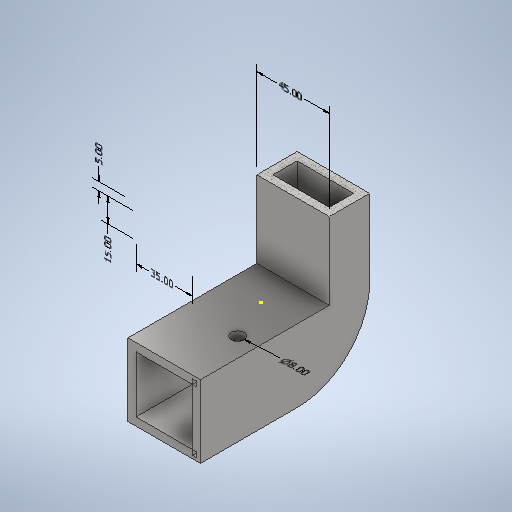
# Autodesk Inventor part: Part2
Saved by Autodesk Inventor 2025.4 (Build 294407000, 407)
## iProperties
Created: 2026-03-03
Part Number: Part2
Material: Iron, Malleable
Document SubType Name: Modeling
Designer: Amir
Density: 7.15 g/cm^3
Appearance: Semi-Polished
Author: Amir
Autodesk Inventor part; units mm, degrees
ref_plane "YZ Plane" through (0, 0, 0) normal (1, 0, 0) x (0, 1, 0)
ref_plane "XZ Plane" through (0, 0, 0) normal (0, 1, 0) x (-1, 0, 0)
ref_plane "XY Plane" through (0, 0, 0) normal (0, 0, 1) x (1, 0, 0)
sketch "Sketch1" plane through (0, 0, 0) normal (0, 0, 1) x (1, 0, 0)
  line L0 (-22.5, -22.5) -> (22.5, -22.5)
  line L1 (22.5, -22.5) -> (22.5, 22.5)
  line L2 (22.5, 22.5) -> (-22.5, 22.5)
  line L3 (-22.5, 22.5) -> (-22.5, -22.5)
  line L4 (-22.5, -22.5) -> (22.5, 22.5) construction
  line L5 (22.5, -22.5) -> (-22.5, 22.5) construction
  line L6 (-17.5, -17.5) -> (17.5, -17.5)
  line L7 (17.5, -17.5) -> (17.5, 17.5)
  line L8 (17.5, 17.5) -> (-17.5, 17.5)
  line L9 (-17.5, 17.5) -> (-17.5, -17.5)
  line L10 (-17.5, -17.5) -> (17.5, 17.5) construction
  line L11 (17.5, -17.5) -> (-17.5, 17.5) construction
  line L12 (-22.5, 17.5) -> (22.5, 17.5)
  point P0 (0, 0)
  dimension "d0" = 45
  dimension "d20" = 5
  dimension "d21" = 5
  constraints: 26 end point, 4 midpoint, 4 parallel, 4 point on line, 2 horizontal, 2 perpendicular
  measures "d0" distance of L2.end L1.end
  measures "d20" distance between parallel lines of L2 L8
  measures "d21" distance between parallel lines of L1 L7
extrude "Extrusion1" add sketch "Sketch1" along normal blind 60 contours L3 L12 L9 L6 L7 L1 L0 | L3 L2 L1 L12 L8
sketch "Sketch2" plane through (0, 0, 0) normal (0, 0, -1) x (-1, 0, 0)
  line L0 (17.5, -17.5) -> (17.5, 17.5) projected
  line L1 (-17.5, -17.5) -> (17.5, -17.5)
  line L2 (17.5, -17.5) -> (17.5, 17.5)
  line L3 (17.5, 17.5) -> (-17.5, 17.5)
  line L4 (-17.5, 17.5) -> (-17.5, -17.5)
  line L5 (-17.5, -17.5) -> (17.5, 17.5) construction
  line L6 (17.5, -17.5) -> (-17.5, 17.5) construction
  line L7 (-22.5, 22.5) -> (22.5, 22.5) projected
  line L8 (-22.5, -22.5) -> (22.5, -22.5)
  line L9 (22.5, -22.5) -> (22.5, 22.5)
  line L10 (22.5, 22.5) -> (-22.5, 22.5)
  line L11 (-22.5, 22.5) -> (-22.5, -22.5)
  line L12 (-22.5, -22.5) -> (22.5, 22.5) construction
  line L13 (22.5, -22.5) -> (-22.5, 22.5) construction
  line L14 (-39.1057, 22.5) -> (57.4203, 22.5)
  point P0 (0, 0)
  dimension "d18" = 5
  dimension "d19" = 5
  constraints: 26 end point, 4 midpoint, 4 parallel, 2 horizontal, 2 perpendicular, 1 point on line
  measures "d18" distance between parallel lines of L8 L1
  measures "d19" distance between parallel lines of L11 L4
revolve "Revolution1" add sketch "Sketch2" angle 90 about axis through (39.1057, 22.5, 0) along (1, 0, 0)
sketch "Sketch3" plane through (-22.5, 22.5, 60) normal (0, 1, 0) x (1, 0, 0)
  line L0 (5, 65) -> (5, 100) projected
  line L1 (40, 85) -> (5, 85)
  line L2 (5, 85) -> (5, 100)
  line L3 (5, 100) -> (40, 100)
  line L4 (35.2339, 98.1928) -> (5, 100) construction
  line L5 (5, 85) -> (35.2339, 113.1928) construction
  line L6 (0, 60) -> (0, 105) projected
  line L7 (45, 80) -> (0, 80)
  line L8 (0, 80) -> (0, 105)
  line L9 (0, 105) -> (45, 105)
  line L10 (40.2339, 93.1928) -> (0, 105) construction
  line L11 (0, 80) -> (45, 122.7171) construction
  line L12 (40, 100) -> (40, 65) projected
  line L13 (40, 100) -> (40, 85)
  line L14 (45, 105) -> (45, 0) projected
  line L15 (45, 105) -> (45, 80)
  point P0 (22.5, 60)
  point P1 (20.117, 99.0964)
  point P2 (43.816, 121.1954)
  point P3 (20.117, 99.0964)
  point P4 (0, 80)
  point P5 (5, 85)
  dimension "d17" = 15
  constraints: 24 end point, 7 point on line, 4 midpoint, 2 horizontal, 2 parallel, 2 perpendicular
  measures "d17" distance between parallel lines of L3 L1
extrude "Extrusion2" add sketch "Sketch3" along normal blind 50
extrude "Extrusion4" add sketch "Sketch1" against normal blind 25 contours L3 L2 L1 L12 L8
extrude "Extrusion5" cut sketch "Sketch3" along normal blind 75.5 contours L0 L3 L12 L1
sketch "Sketch10" plane through (-22.5, 72.5, 60) normal (0, 1, 0) x (1, 0, 0)
  line L0 (45, 105) -> (0, 105)
  line L1 (0, 105) -> (0, 80)
  line L2 (0, 80) -> (45, 80)
  line L3 (45, 80) -> (45, 105)
  line L4 (5, 100) -> (40, 100) projected
  line L5 (40, 85) -> (5, 85) projected
  line L6 (40, 100) -> (5, 100)
  line L7 (5, 100) -> (5, 85)
  line L8 (5, 85) -> (40, 85)
  line L9 (40, 85) -> (40, 100)
  line L10 (-3.6161, 80) -> (47.5585, 80)
  constraints: 18 end point, 4 parallel, 2 horizontal, 2 perpendicular, 1 point on line
revolve "Revolution3" add sketch "Sketch10" angle 90 about axis through (-26.1161, 72.5, -20) along (1, 0, 0)
sketch "Sketch11" plane through (-22.5, 22.5, -20) normal (0, 0, 1) x (1, 0, 0)
  line L0 (45, 75) -> (0, 75) projected
  line L1 (45, 50) -> (0, 50) projected
  line L2 (45, 75) -> (0, 75)
  line L3 (0, 75) -> (0, 50)
  line L4 (0, 50) -> (45, 50)
  line L5 (45, 50) -> (45, 75)
  line L6 (40, 70) -> (40, 55) projected
  line L7 (40, 55) -> (5, 55) projected
  line L8 (40, 70) -> (5, 70)
  line L9 (5, 70) -> (5, 55)
  line L10 (5, 55) -> (40, 55)
  line L11 (40, 55) -> (40, 70)
  point P0 (22.5, -22.5)
  dimension "d68" = 15
  constraints: 16 end point, 4 parallel, 2 horizontal, 2 perpendicular
  measures "d68" distance between parallel lines of L7 L8
extrude "Extrusion8" add sketch "Sketch11" along normal blind 80
sketch "Sketch12" plane through (-22.5, 22.5, 60) normal (0, 1, 0) x (1, 0, 0)
  point P0 (22.5, 60)
sketch "Sketch13" plane through (0, 0, 60) normal (0, 0, 1) x (1, 0, 0)
  line L0 (17.5, 17.5) -> (17.5, -17.5) projected
  line L1 (17.5, 17.5) -> (19.8638, 17.5)
  line L2 (19.8638, 17.5) -> (19.8638, 20.41)
  line L3 (19.8638, 20.41) -> (17.5, 20.41)
  line L4 (17.5, 20.41) -> (17.5, 17.5)
  line L5 (17.5, -17.5) -> (19.8638, -17.5)
  line L6 (19.8638, -17.5) -> (19.8638, -20.6538)
  line L7 (19.8638, -20.6538) -> (17.5, -20.6538)
  line L8 (17.5, -20.6538) -> (17.5, -17.5)
  point P0 (0, 0)
  constraints: 16 end point, 4 parallel, 2 horizontal, 2 perpendicular, 1 point on line
extrude "Extrusion9" cut sketch "Sketch13" against normal blind 80.25
sketch "Sketch14" plane through (-22.5, 22.5, 60) normal (0, 1, 0) x (1, 0, 0)
  circle A0 centre (33.1575, 35) radius 4
  line L0 (45, 0) -> (0, 0) projected
  point P0 (22.5, 60)
  dimension "d72" = 8
  dimension "d73" = 35
  constraints: 1 centre point
  measures "d72" diameter of A0
  measures "d73" distance from line of L0 A0.centre
extrude "Extrusion10" cut sketch "Sketch14" against normal blind 28.5
body "Solid1"
